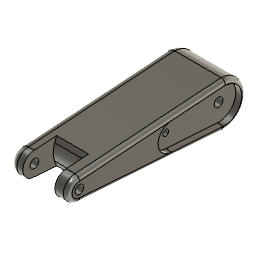
Assieme (Autodesk Fusion 360 archive; units mm, degrees)
design "Braccio cort"
Autodesk Fusion 360 part; units mm, degrees
sketch "Sketch1" plane through (0, 0, 0) normal (1, 0, 0) x (0, 1, 0)
  circle A0 centre (0, 0) radius 5.95
  line L0 (0, 0) -> (-18.2, 0)
  circle A1 centre (-18.2, 0) radius 4.7
  line L1 (-18.2, 4.7) -> (-0.412348, 5.935694)
  line L2 (-18.2, -4.7) -> (-0.412348, -5.935694)
  line L3 (0, 0) -> (-50, 0)
  circle A2 centre (-50, 0) radius 1.5
  circle A3 centre (0, 0) radius 7.5
  circle A4 centre (-50, 0) radius 4
  line L4 (-50.000001, 4) -> (0.297212, 7.494109)
  line L5 (-50.000001, -4) -> (-0.52648, -7.481498)
  circle A5 centre (0, 0) radius 1.5
  dimension "d1" = 11.9
  dimension "d2" = 18.2
  dimension "d3" = 9.4
  dimension "d4" = 50
  dimension "d5" = 3
  dimension "d6" = 15
  dimension "d7" = 8
  dimension "d12" = 3
  constraint coincident A0.centre L0.start
  constraint horizontal L0
  constraint coincident L0.end A1.centre
  constraint coincident A1 L1.start
  constraint tangent A0 L1
  constraint coincident A1 L2.start
  constraint tangent A0 L2
  constraint parallel L0 L3
  constraint coincident L3.end A2.centre
  constraint concentric A0 A3
  constraint concentric A2 A4
  constraint parallel L1 L4
  constraint tangent A3 L5
  constraint concentric A3 A5
  measures "d1" diameter of A0
  measures "d2" distance of A0.centre L0.end
  measures "d3" diameter of A1
  measures "d4" distance of A0.centre L3.end
  measures "d5" diameter of A2
  measures "d6" diameter of A3
  measures "d7" diameter of A4
  measures "d12" diameter of A5
extrude "Extrude1" add sketch "Sketch1" against normal blind 20 contours A0 | A0 L1 L2 A3 L4 | A0 L0 L1 L3 A3 | A0 L0 L2 L3 A3 | L0 A1 L1 L3 A3 | A1 L1 L3 A3 A4 L4 | A1 L2 L3 A3 A4 L5 | L0 A1 L2 L3 A3 | L0 A1 L3 | L0 A1 L3 | A4 | A2 | A5 picked at (0.057913, 4.454197) picked at (-0.481904, 6.936944) picked at (-4.913133, 4.943319) picked at (-4.913133, -4.943319) picked at (-9.491083, 0.574667) picked at (-23.269385, 5.029406) picked at (-23.455372, -5.333731) picked at (-9.491083, -0.574667) picked at (-17.97704, 3.117387) picked at (-21.317387, -0.22296) picked at (-50.236089, -3.150376) picked at (-49.655688, 0.192709) picked at (0.715636, -0.549431)
extrude "Extrude2" cut sketch "Sketch1" against normal blind 2.05 contours A0 | A0 L0 L1 L3 A3 | A0 L0 L2 L3 A3 | L0 A1 L1 L3 A3 | L0 A1 L2 L3 A3 | L0 A1 L3 | L0 A1 L3 | A5 picked at (0.057913, 4.454197) picked at (-4.913133, 4.943319) picked at (-4.913133, -4.943319) picked at (-9.491083, 0.574667) picked at (-9.491083, -0.574667) picked at (-17.97704, 3.117387) picked at (-21.317387, -0.22296) picked at (0.715636, -0.549431)
extrude "Extrude3" cut sketch "Sketch1" against normal through all contours A2 | A5 picked at (-49.655688, 0.192709) picked at (0.715636, -0.549431)
sketch "Sketch2" plane through (-20, 0, 0) normal (-1, 0, 0) x (0, -1, 0)
  arc A0 (50.000001, -4) -> (50.000001, 4) centre (50, 0) ccw
  line L0 (50.000001, 4) -> (-0.297212, 7.494109)
  arc A1 (-0.297212, 7.494109) -> (0.52648, -7.481498) centre (0, 0) ccw
  line L1 (0.52648, -7.481498) -> (50.000001, -4)
  circle A2 centre (0, 0) radius 3
  circle A3 centre (0, 0) radius 1.5
  circle A4 centre (50, 0) radius 1.5
  dimension "d15" = 6
  measures "d15" diameter of A2
extrude "Extrude4" cut sketch "Sketch2" against normal blind 10 contours A2 | A3 picked at (2.488831, -0.149042) picked at (0.56701, -0.538293)
sketch "Sketch3" plane through (0, 0, 0) normal (1, 0, 0) x (0, 1, 0)
  circle A0 centre (-50.000001, 0) radius 6
  line L0 (-44.000001, 7) -> (-56.000001, 7)
  line L1 (-56.000001, 7) -> (-56.000001, -7)
  line L2 (-56.000001, -7) -> (-44.000001, -7)
  line L3 (-44.000001, -7) -> (-44.000001, 7)
  line L4 (-44.000001, 7) -> (-56.000001, -7) construction
  line L5 (-56.000001, 7) -> (-44.000001, -7) construction
  line L6 (-44.000001, 0) -> (-40.579799, 9.396926)
  line L7 (-44.000001, 0) -> (-34.000001, 0) construction
  line L8 (-44.000001, 7) -> (-39.000001, 7)
  line L9 (-50.000001, 0) -> (-39.000001, 0)
  line L10 (-44.000001, -7) -> (-39.000001, -7)
  line L11 (-44.000001, 0) -> (-40.579799, -9.396926)
  point P0 (-50.000001, 0)
  dimension "d18" = 12
  dimension "d22" = 70
  dimension "d23" = 10
  constraint horizontal L0
  constraint perpendicular L0 L1
  constraint parallel L0 L2
  constraint parallel L1 L3
  constraint horizontal L7
  constraint perpendicular L3 L8
  measures "d18" diameter of A0
  measures "d22" angle of L6 L7
extrude "Extrude5" cut sketch "Sketch3" along normal mid plane 11 from surface at -10 contours A0 | A0 L1 L2 L3 | L3 L10 L11 | A0 L0 L1 L3 | L3 L6 L8 picked at (-50.136181, 1.817196) picked at (-50.149461, -6.661074) picked at (-43.150737, -4.666667) picked at (-50.149461, 6.661074) picked at (-43.150737, 4.666667)
sketch "Sketch4" plane through (-2.05, 0, 0) normal (1, 0, 0) x (0, 1, 0)
  circle A0 centre (0, 0) radius 1.5
  arc A1 (-18.2, 4.7) -> (-18.2, -4.7) centre (-18.2, 0) ccw
  line L0 (-18.2, -4.7) -> (-0.412348, -5.935694)
  arc A2 (-0.412348, -5.935694) -> (-0.412348, 5.935694) centre (0, 0) ccw
  line L1 (-0.412348, 5.935694) -> (-18.2, 4.7)
  circle A3 centre (-18.2, 0) radius 4.7
  circle A4 centre (-18.2, 0) radius 1
  dimension "d24" = 2
  constraint concentric A1 A3
  constraint concentric A3 A4
  measures "d24" diameter of A4
extrude "Extrude6" cut sketch "Sketch4" against normal blind 9 contours A4 picked at (-18.12804, 0.310291)
fillet "Fillet1" radius 8 1 edges at (-10, -44.000001, 0)
fillet "Fillet2" radius 2.5 4 edges at (-20, -24.851395, 5.747054) (-20, 7.488681, -0.411894) (-20, -25.26324, -5.740749) (-20, -54, 0)
fillet "Fillet2" radius 1.5 4 edges at (0, -24.851395, 5.747054) (0, -25.26324, -5.740749) (0, 7.488681, -0.411894) (0, -54, 0)

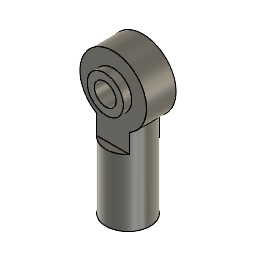
design "M3 angolare"
Autodesk Fusion 360 part; units mm, degrees
sketch "Sketch1" plane through (0, 0, 0) normal (0, 0, 1) x (1, 0, 0)
  circle A0 centre (0, 0) radius 3
  dimension "d6" = 6
  constraint coincident A0.centre origin
  measures "d6" diameter of A0
extrude "Extrude1" add sketch "Sketch1" along normal blind 15.5 makes body 1
sketch "Sketch3" plane through (0, 0, 0) normal (0, 1, 0) x (1, 0, 0)
  line L0 (0, 0) -> (0, -15.5)
  circle A0 centre (0, -15.5) radius 4.5
  circle A1 centre (0, -15.5) radius 2.5
  dimension "d5" = 9
  dimension "d9" = 5
  constraint coincident L0.start origin
  constraint vertical L0
  constraint coincident L0.end A0.centre
  constraint concentric A0 A1
  measures "d5" diameter of A0
  measures "d9" diameter of A1
extrude "Extrude2" add sketch "Sketch3" along normal mid plane 6 contours A0 | A1 bodies 1
extrude "Extrude3" cut sketch "Sketch3" along normal mid plane 6 contours A1 bodies 1
sketch "Sketch4" plane through (0, 0, 0) normal (1, 0, 0) x (0, 1, 0)
  line L0 (0, 20) -> (2, 20)
  line L1 (2, 20) -> (-2, 20)
  line L2 (-2, 20) -> (-2, 9)
  line L3 (-2, 9) -> (2, 9)
  line L4 (2, 9) -> (2, 20)
  line L5 (-3, 20) -> (3, 20)
  line L6 (3, 20) -> (3, 9)
  line L7 (3, 9) -> (-3, 9)
  line L8 (-3, 9) -> (-3, 20)
  dimension "d12" = 2
  dimension "d13" = 4
  dimension "d14" = 11
  constraint horizontal L0
  constraint horizontal L1
  constraint vertical L2
  constraint horizontal L3
  constraint vertical L4
  constraint horizontal L5
  constraint vertical L6
  constraint horizontal L7
  constraint vertical L8
  measures "d12" distance of L0.start L0.end
  measures "d13" distance of L0.end L1.end
  measures "d14" distance of L0.end L3.end
extrude "Extrude4" cut sketch "Sketch4" along normal mid plane 10 contours L4 L5 L6 L7 | L2 L5 L7 L8 bodies 1
sketch "Sketch5" plane through (0, 0, 0) normal (1, 0, 0) x (0, 1, 0)
  circle A0 centre (-10.5, -7) radius 2.5
  circle A1 centre (-10.5, -7) radius 1.5
  dimension "d19" = 5
  dimension "d20" = 3
  constraint concentric A0 A1
  measures "d19" diameter of A0
  measures "d20" diameter of A1
extrude "Extrude5" add sketch "Sketch5" along normal blind 6 separate body makes body 2
copy_body "Body->Comp1" bodies 1 removing the originals makes body 3 in component "Component"
copy_body "Body->Comp2" bodies 2 removing the originals makes body 4 in component "Component'"
component "Component" placed x (1, 0, 0) y (0, 1, 0) z (0, 0, 1) at (0, 0, 0)
component "Component'" placed x (0, -1, 0) y (1, 0, 0) z (0, 0, 1) at (10.5, 3, 22.5)
component "M3 angolare v1" placed x (1, 0, 0) y (0, 1, 0) z (0, 0, 1) at (0, 0, 0) in component "Component"
equation "d1 = 20 mm - 4.5 mm"

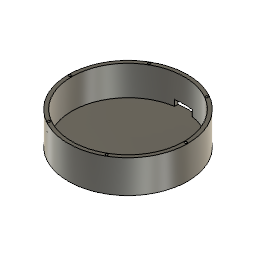
design "Base"
Autodesk Fusion 360 part; units mm, degrees
sketch "Sketch1" plane through (0, 0, 0) normal (0, 0, 1) x (1, 0, 0)
  circle A0 centre (0, 0) radius 100
  circle A1 centre (0, 0) radius 94
  dimension "d1" = 200
  dimension "d2" = -6
  constraint coincident A0.centre A1.centre
  measures "d1" diameter of A0
extrude "Extrude1" add sketch "Sketch1" along normal blind 50
sketch "Sketch2" plane through (0, 0, 50) normal (0, 0, 1) x (-1, 0, 0)
  circle A0 centre (0, 0) radius 94
  circle A1 centre (0, 0) radius 100
  circle A2 centre (0, 0) radius 94
  circle A3 centre (0, 0) radius 100
  circle A4 centre (0, 0) radius 97
  line L0 (0, 0) -> (115, 0)
  circle A5 centre (97, 0) radius 2
  dimension "d7" = 194
  dimension "d8" = 200
  dimension "d9" = 188
  dimension "d10" = 4
  constraint concentric A0 A2
  constraint coincident A0.centre A1.centre
  constraint horizontal L0
  constraint coincident A4 A5.centre
  constraint coincident L0 A5.centre
  measures "d7" diameter of A4
  measures "d8" diameter of A3
  measures "d9" diameter of A2
  measures "d10" diameter of A5
extrude "Extrude2" cut sketch "Sketch2" against normal blind 15 contours A4 L0 A5 | A4 L0 A5 | A4 L0 A5 | A4 L0 A5
pattern_circular "C-Pattern1" count 6 over 360 about axis through (0, 0, 1.75) along (0, 0, 1) of "Extrude2"
sketch "Sketch3" plane through (0, 0, 0) normal (0, 0, -1) x (1, 0, 0)
  circle A0 centre (0, 0) radius 94
  circle A1 centre (0, 0) radius 100
  circle A2 centre (0, 0) radius 100
  constraint concentric A0 A2
extrude "Extrude3" add sketch "Sketch3" along normal blind 5 contours A0 | A1 A2
sketch "Sketch4" plane through (0, 0, 0) normal (0, 1, 0) x (1, 0, 0)
  line L0 (0, 0) -> (15, 0)
  line L1 (15, 0) -> (15, -10)
  line L2 (15, -10) -> (0, -10)
  line L3 (0, -10) -> (0, 0)
  line L4 (0, 0) -> (-15, 0)
  line L5 (-15, 0) -> (-15, -10)
  line L6 (-15, -10) -> (0, -10)
  line L7 (0, -10) -> (0, 0)
  dimension "d17" = 15
  dimension "d18" = 10
  dimension "d19" = 10
  constraint horizontal L0
  constraint vertical L1
  constraint horizontal L2
  constraint vertical L3
  constraint coincident L0.start L3.end
  constraint horizontal L4
  constraint vertical L5
  constraint horizontal L6
  constraint vertical L7
  measures "d17" distance of L0.start L0.end
  measures "d18" distance of L0.start L2.end
  measures "d19" distance of L0.start L2.end
extrude "Extrude4" cut sketch "Sketch4" along normal blind 100
equation "d7 = d9 + ( ( d8 - d9 ) * 0.5 )"

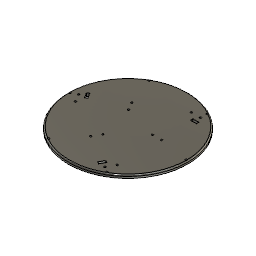
design "Senza titolo"
Autodesk Fusion 360 part; units mm, degrees
sketch "Schizzo1" plane through (0, 0, 0) normal (0, 0, 1) x (1, 0, 0)
  line L0 (0, 0) -> (0, 50)
  line L1 (0, 50) -> (0, 60.7)
  line L2 (0, 60.7) -> (37, 60.7)
  line L3 (37, 60.7) -> (37, 20.7)
  line L4 (37, 20.7) -> (0, 20.7)
  line L5 (0, 20.7) -> (0, 60.7)
  line L6 (-52.5677, -30.35) -> (-71.0677, 1.6929)
  line L7 (0, 0) -> (-43.3013, -25)
  line L8 (-36.4267, 21.6929) -> (-17.9267, -10.35)
  line L9 (-71.0677, 1.6929) -> (-36.4267, 21.6929)
  line L10 (-43.3013, -25) -> (-52.5677, -30.35)
  line L11 (-17.9267, -10.35) -> (-52.5677, -30.35)
  line L12 (52.5677, -30.35) -> (34.0677, -62.3929)
  line L13 (0, 0) -> (43.3013, -25)
  line L14 (-0.5733, -42.3929) -> (17.9267, -10.35)
  line L15 (34.0677, -62.3929) -> (-0.5733, -42.3929)
  line L16 (43.3013, -25) -> (52.5677, -30.35)
  line L17 (17.9267, -10.35) -> (52.5677, -30.35)
  circle A0 centre (0, 0) radius 100
  dimension "d1" = 50
  dimension "d2" = 10.7
  dimension "d3" = 37
  dimension "d4" = 40
  dimension "d6" = 360
  dimension "d7" = 200
  constraint coincident L0.start L7.start
  constraint vertical L0
  constraint parallel L0 L1
  constraint horizontal L2
  constraint vertical L3
  constraint horizontal L4
  constraint vertical L5
  measures "d1" distance of L0.start L0.end
  measures "d2" distance of L0.end L1.end
  measures "d3" distance of L1.end L2.end
  measures "d4" distance of L1.end L4.end
  measures "d7" diameter of A0
extrude "Estrusione1" add sketch "Schizzo1" along normal blind 10 contours L0 L1 L2 L3 L4 L5 | L6 L7 L8 L9 L10 L11 | L12 L13 L14 L15 L16 L17 | A0
sketch "Schizzo2" plane through (0, 0, 10) normal (0, 0, 1) x (-1, 0, 0)
  circle A0 centre (0, 0) radius 100
  line L0 (0, 0) -> (0, -50)
  line L1 (0, -50) -> (-32.95, -50)
  line L2 (-32.95, -50) -> (-32.95, -73.2)
  line L3 (-32.95, -73.2) -> (-47.95, -73.2)
  line L4 (-47.95, -73.2) -> (-47.95, -8.2)
  line L5 (-47.95, -8.2) -> (-32.95, -8.2)
  line L6 (-32.95, -8.2) -> (-32.95, -73.2)
  circle A1 centre (-32.95, -73.2) radius 1.5
  circle A2 centre (-32.95, -8.2) radius 1.5
  circle A3 centre (-47.95, -73.2) radius 1.5
  circle A4 centre (-47.95, -8.2) radius 1.5
  dimension "d33" = 50
  dimension "d34" = 32.95
  dimension "d35" = 23.2
  dimension "d36" = 15
  dimension "d37" = 65
  dimension "d38" = 3
  dimension "d39" = 3
  dimension "d40" = 3
  dimension "d41" = 3
  constraint coincident A0.centre L0.start
  constraint vertical L0
  constraint perpendicular L0 L1
  constraint perpendicular L1 L2
  constraint horizontal L3
  constraint vertical L4
  constraint horizontal L5
  constraint vertical L6
  constraint coincident L2.end L3.start
  constraint coincident L5.end L6.start
  constraint coincident L3.end L4.start
  constraint coincident L4.end L5.start
  measures "d33" distance of A0.centre L0.end
  measures "d34" distance of L0.end L1.end
  measures "d35" distance of L1.end L2.end
  measures "d36" distance of L2.end L3.end
  measures "d37" distance of L2.end L5.end
  measures "d38" diameter of A1
  measures "d39" diameter of A2
  measures "d40" diameter of A3
  measures "d41" diameter of A4
extrude "Extrude4" cut sketch "Schizzo2" against normal blind 60 contours L2 L3 L6 A1 | L2 L3 L6 A1 | L5 L6 A2 | L5 L6 A2 | L3 L4 A3 | L3 L4 A3 | L4 L5 A4 | L4 L5 A4
pattern_circular "C-Pattern2" count 3 over 360 about axis through (0, 0, 1.75) along (0, 0, 1) of "Extrude4"
sketch "Sketch4" plane through (0, 0, 10) normal (0, 0, 1) x (-1, 0, 0)
  circle A0 centre (0, 0) radius 100
  circle A1 centre (-32.95, -8.2) radius 1.5
  circle A2 centre (-32.95, -73.2) radius 1.5
  circle A3 centre (-47.95, -8.2) radius 1.5
  circle A4 centre (-47.95, -73.2) radius 1.5
  circle A5 centre (31.0764, -37.4259) radius 1.5
  circle A6 centre (79.8681, 8.0645) radius 1.5
  circle A7 centre (87.3681, -4.9259) radius 1.5
  circle A8 centre (23.5764, -24.4355) radius 1.5
  circle A9 centre (16.8736, 45.6259) radius 1.5
  circle A10 centre (-46.9181, 65.1355) radius 1.5
  circle A11 centre (-39.4181, 78.1259) radius 1.5
  circle A12 centre (9.3736, 32.6355) radius 1.5
  line L0 (-38.5766, 79.3677) -> (-31.6381, 75.3854)
  line L1 (-31.6381, 75.3854) -> (-34.6248, 70.1816)
  line L2 (-34.6248, 70.1816) -> (-31.1556, 68.1905)
  line L3 (-31.6381, 75.3854) -> (-28.1689, 73.3943)
  line L4 (-28.1689, 73.3943) -> (-31.1556, 68.1905)
  line L5 (-28.1689, 73.3943) -> (-26.1778, 76.8635)
  line L6 (-31.6381, 75.3854) -> (-29.647, 78.8547)
  line L7 (-29.647, 78.8547) -> (-26.1778, 76.8635)
  dimension "d46" = 8
  dimension "d47" = 6
  dimension "d48" = 4
  dimension "d49" = 4
  dimension "d54" = 4
  dimension "d55" = 4
  constraint coincident A11 L0.start
  constraint perpendicular L0 L1
  constraint perpendicular L1 L2
  constraint perpendicular L1 L3
  constraint perpendicular L3 L5
  constraint perpendicular L3 L6
  measures "d46" distance of L0.start L0.end
  measures "d47" distance of L0.end L1.end
  measures "d48" distance of L1.end L2.end
  measures "d49" distance of L0.end L3.end
  measures "d54" distance of L3.end L5.end
  measures "d55" distance of L0.end L6.end
extrude "Extrude5" cut sketch "Sketch4" against normal blind 40 contours L1 L2 L3 L4 | L3 L5 L6 L7
pattern_circular "C-Pattern3" count 3 over 360 about axis through (0, 0, -200) along (0, 0, 1) of "Extrude5"
extrude "Extrude6" cut 1 faces at (23.6749, -29.9689, 0) along direction (0, 0, 1) blind 5
sketch "Sketch5" plane through (0, 0, 10) normal (0, 0, 1) x (-1, 0, 0)
  line L0 (-31.1556, 68.1905) -> (-34.6248, 70.1816)
  line L1 (-34.6248, 70.1816) -> (-29.647, 78.8547)
  line L2 (-29.647, 78.8547) -> (-26.1778, 76.8635)
  line L3 (-26.1778, 76.8635) -> (-31.1556, 68.1905)
  circle A0 centre (0, 0) radius 100
  circle A1 centre (-32.95, -8.2) radius 1.5
  circle A2 centre (-32.95, -73.2) radius 1.5
  circle A3 centre (-47.95, -8.2) radius 1.5
  circle A4 centre (-47.95, -73.2) radius 1.5
  circle A5 centre (31.0764, -37.4259) radius 1.5
  circle A6 centre (79.8681, 8.0645) radius 1.5
  circle A7 centre (87.3681, -4.9259) radius 1.5
  circle A8 centre (23.5764, -24.4355) radius 1.5
  circle A9 centre (16.8736, 45.6259) radius 1.5
  circle A10 centre (-46.9181, 65.1355) radius 1.5
  circle A11 centre (-39.4181, 78.1259) radius 1.5
  circle A12 centre (9.3736, 32.6355) radius 1.5
  line L4 (-43.4769, -61.0768) -> (-43.4667, -65.0768)
  line L5 (-43.4667, -65.0768) -> (-53.4666, -65.1024)
  line L6 (-53.4666, -65.1024) -> (-53.4769, -61.1024)
  line L7 (-53.4769, -61.1024) -> (-43.4769, -61.0768)
  line L8 (74.6325, -7.1137) -> (78.0914, -5.1049)
  line L9 (78.0914, -5.1049) -> (83.1136, -13.7523)
  line L10 (83.1136, -13.7523) -> (79.6547, -15.7611)
  line L11 (79.6547, -15.7611) -> (74.6325, -7.1137)
  circle A13 centre (0, 0) radius 97
  line L12 (0, 0) -> (97, 0)
  circle A14 centre (97, 0) radius 1.5
  dimension "d60" = 194
  dimension "d61" = 3
  constraint coincident A0.centre A13.centre
  constraint coincident A13 L12.end
  constraint horizontal L12
  constraint coincident L12.end A14.centre
  measures "d60" diameter of A13
  measures "d61" diameter of A14
extrude "Extrude7" cut sketch "Sketch5" against normal blind 9.5 contours A13 L12 A14 | A13 A14 | A13 L12 A14 picked at (97.4791, 0.3082)
pattern_circular "C-Pattern4" count 6 over 360 about axis through (0, 0, 1.75) along (0, 0, 1) of "Extrude7"
fillet "Fillet2" radius 2 1 edges at (-93.2327, -36.1615, 10)
equation "d34 = 25 mm + 2.95 mm + 5 mm"
equation "d48 = d49"

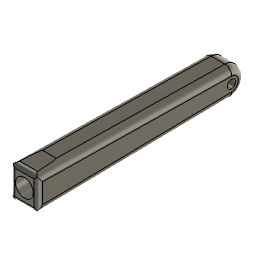
design "Braccio lungo"
Autodesk Fusion 360 part; units mm, degrees
sketch "Sketch1" plane through (0, 0, 0) normal (1, 0, 0) x (0, 1, 0)
  circle A0 centre (0, 0) radius 5
  circle A1 centre (0, 0) radius 1.5
  line L0 (0, 0) -> (-61, 0)
  line L1 (-61, -3.25) -> (-61, 3.25)
  line L2 (-61, -6) -> (-61, 6)
  line L3 (-61, 6) -> (0.081901, 4.999329)
  line L4 (-61, -6) -> (0.081901, -4.999329)
  dimension "d1" = 10
  dimension "d2" = 3
  dimension "d3" = 61
  dimension "d4" = 6.5
  dimension "d5" = 12
  constraint coincident A0.centre A1.centre
  constraint horizontal L0
  constraint midpoint L0.end L1
  constraint perpendicular L0 L1
  constraint midpoint L0.end L2
  constraint perpendicular L0 L2
  constraint tangent A0 L3
  constraint tangent A0 L4
  measures "d1" diameter of A0
  measures "d2" diameter of A1
  measures "d3" distance of A0.centre L0.end
  measures "d4" distance of L1.start L1.end
  measures "d5" distance of L2.start L2.end
extrude "Extrude1" add sketch "Sketch1" along normal mid plane 10 contours A0 | A0 L0 L1 L2 L3 | A0 L0 L1 L2 L4 picked at (-0.222664, -3.818097) picked at (-42.333333, 1.083333) picked at (-42.333333, -1.083333)
ref_plane "WorkPlane1" through (0, -61, 0) normal (0, 1, 0) x (0, 0, 1)
sketch "Sketch2" plane through (0, -61, 0) normal (0, 1, 0) x (1, 0, 0)
  circle A0 centre (0, 0) radius 3.25
  circle A1 centre (0, 0) radius 6
  line L0 (-5, -6) -> (5, -6)
  line L1 (5, -6) -> (5, 6)
  line L2 (5, 6) -> (-5, 6)
  line L3 (-5, 6) -> (-5, -6)
  line L4 (-5, -6) -> (5, 6) construction
  line L5 (5, -6) -> (-5, 6) construction
  dimension "d9" = 6.5
  dimension "d10" = 12
  constraint coincident A0.centre A1.centre
  constraint concentric A0 A1
  constraint horizontal L0
  constraint perpendicular L0 L1
  constraint parallel L0 L2
  constraint parallel L1 L3
  constraint coincident L4 A0.centre
  constraint coincident L5 A0.centre
  measures "d9" diameter of A0
  measures "d10" diameter of A1
extrude "Extrude2" add sketch "Sketch2" against normal blind 9 contours A1 L1 L3 | A1 L1 L2 | A1 L0 L1 | A1 L2 L3 | A1 L0 L3 picked at (4.416667, 0) picked at (4.027994, 5.216371) picked at (4.027994, -5.216371) picked at (-4.027994, 5.216371) picked at (-4.027994, -5.216371)
sketch "Sketch3" plane through (0, -61, 0) normal (0, -1, 0) x (1, 0, 0)
  circle A0 centre (0, 0) radius 3.25
  circle A1 centre (0, 0) radius 1.5
  dimension "d13" = 3
  constraint coincident A0.centre A1.centre
  measures "d13" diameter of A1
extrude "Extrude3" cut sketch "Sketch3" against normal blind 6 contours A1 picked at (0.56701, -0.538293)
sketch "Sketch4" plane through (-5, 0, 0) normal (-1, 0, 0) x (0, -1, 0)
  circle A0 centre (0, 0) radius 1.5
  line L0 (61, 6) -> (-0.081901, 4.999329)
  arc A1 (-0.081901, 4.999329) -> (-0.081901, -4.999329) centre (0, 0) ccw
  line L1 (-0.081901, -4.999329) -> (61, -6)
  line L2 (61, -6) -> (70, -6)
  line L3 (70, -6) -> (70, 6)
  line L4 (70, 6) -> (61, 6)
  line L5 (70, 0) -> (57, 0)
  line L6 (57, 0) -> (57, 3)
  line L7 (57, 3) -> (32, 3)
  line L8 (32, 3) -> (32, -3)
  line L9 (32, -3) -> (57, -3)
  line L10 (57, -3) -> (57, 3)
  dimension "d16" = 13
  dimension "d17" = 3
  dimension "d18" = 25
  dimension "d19" = 6
  constraint midpoint L3 L5.start
  constraint perpendicular L3 L5
  constraint perpendicular L5 L6
  constraint horizontal L7
  constraint vertical L8
  constraint horizontal L9
  constraint vertical L10
  measures "d16" distance of L5.start L5.end
  measures "d17" distance of L5.end L6.end
  measures "d18" distance of L6.end L7.end
  measures "d19" distance of L6.end L9.end
extrude "Extrude4" cut sketch "Sketch4" against normal blind 7 contours L6 L7 L8 L9 L10 picked at (40.333333, 0)
fillet "Fillet1" radius 1.5 4 edges at (-5, -70, 0) (0, -70, 6) (5, -70, 0) (0, -70, -6)
fillet "Fillet2" radius 2.5 6 edges at (-5, -30.459049, 5.499665) (-5, 5, 0) (-5, -30.459049, -5.499665) (5, -30.459049, -5.499665) (5, 5, 0) (5, -30.459049, 5.499665)
chamfer "Chamfer1" distance 14 distance2 5 1 edges at (-5, -32, 0) measured on face at (-5, -21.833333, 0)
sketch "Sketch5" plane through (2, 0, 0) normal (-1, 0, 0) x (0, -1, 0)
  line L0 (57, -3) -> (57, 3)
  line L1 (57, 3) -> (32, 3)
  line L2 (32, 3) -> (32, -3)
  line L3 (32, -3) -> (57, -3)
  line L4 (57, -3) -> (54, -3)
  line L5 (54, -3) -> (54, 3)
  line L6 (54, 3) -> (57, 3)
  line L7 (57, 3) -> (57, -3)
  dimension "d28" = 3
  dimension "d29" = 6
  constraint horizontal L4
  constraint vertical L5
  constraint horizontal L6
  constraint vertical L7
  constraint coincident L0.start L3.end
  measures "d28" distance of L0.start L4.end
  measures "d29" distance of L0.start L0.end
extrude "Extrude5" cut sketch "Sketch5" against normal blind 1 contours L0 L1 L3 L4 L5 L6 L7 picked at (55, 1)

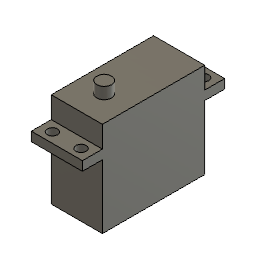
design "Motore"
Autodesk Fusion 360 part; units mm, degrees
sketch "Schizzo1" plane through (0, 0, 0) normal (0, 1, 0) x (1, 0, 0)
  line L0 (0, 0) -> (20, 0)
  line L1 (20, 0) -> (20, 40)
  line L2 (20, 40) -> (0, 40)
  line L3 (0, 40) -> (0, 0)
  dimension "d1" = 20
  dimension "d2" = 40
  constraint horizontal L0
  constraint vertical L1
  constraint horizontal L2
  constraint vertical L3
  constraint coincident L0.start L3.end
  measures "d1" distance of L0.start L0.end
  measures "d2" distance of L0.start L2.end
extrude "Estrusione1" add sketch "Schizzo1" along normal blind 25
sketch "Schizzo2" plane through (0, 25, 0) normal (0, 1, 0) x (-1, 0, 0)
  line L0 (0, -40) -> (0, 0)
  line L1 (0, 0) -> (-20, 0)
  line L2 (-20, 0) -> (-20, -40)
  line L3 (-20, -40) -> (0, -40)
  line L4 (0, -40) -> (0, -47.8)
  line L5 (0, -47.8) -> (-20, -47.8)
  line L6 (-20, -47.8) -> (-20, 7.8)
  line L7 (-20, 7.8) -> (0, 7.8)
  line L8 (0, 7.8) -> (0, -47.8)
  dimension "d5" = 7.8
  dimension "d6" = 55.6
  constraint coincident L0.start L3.end
  constraint perpendicular L3 L4
  constraint horizontal L5
  constraint vertical L6
  constraint horizontal L7
  constraint vertical L8
  measures "d5" distance of L0.start L4.end
  measures "d6" distance of L4.end L7.end
extrude "Estrusione2" add sketch "Schizzo2" along normal blind 3.6
sketch "Schizzo3" plane through (0, 28.6, 0) normal (0, 1, 0) x (-1, 0, 0)
  line L0 (0, 7.8) -> (-20, 7.8)
  line L1 (-20, 7.8) -> (-20, -47.8)
  line L2 (-20, -47.8) -> (0, -47.8)
  line L3 (0, -47.8) -> (0, 7.8)
  line L4 (0, -47.8) -> (-20, -47.8)
  line L5 (-20, -47.8) -> (-20, -40)
  line L6 (-20, -40) -> (0, -40)
  line L7 (0, -40) -> (0, -47.8)
  line L8 (0, 7.8) -> (-20, 7.8)
  line L9 (-20, 7.8) -> (-20, 0)
  line L10 (-20, 0) -> (0, 0)
  line L11 (0, 0) -> (0, 7.8)
  dimension "d9" = 20
  dimension "d10" = 7.8
  dimension "d11" = 7.8
  constraint horizontal L4
  constraint vertical L5
  constraint horizontal L6
  constraint vertical L7
  constraint coincident L2.end L3.start
  constraint horizontal L8
  constraint vertical L9
  constraint horizontal L10
  constraint vertical L11
  constraint coincident L0.start L3.end
  measures "d9" distance of L2.end L1.end
  measures "d10" distance of L2.end L6.end
  measures "d11" distance of L0.start L10.end
extrude "Estrusione3" add sketch "Schizzo3" along normal blind 8.4 contours L1 L3 L6 L10
sketch "Schizzo4" plane through (0, 37, 0) normal (0, 1, 0) x (-1, 0, 0)
  line L0 (-20, -40) -> (0, -40)
  line L1 (0, -40) -> (0, 0)
  line L2 (0, 0) -> (-20, 0)
  line L3 (-20, 0) -> (-20, -40)
  line L4 (-10, 0) -> (-10, -13.6)
  circle A0 centre (-10, -10.7) radius 2.9
  dimension "d14" = 13.6
  dimension "d17" = 5.8
  dimension "d18" = 2.9
  constraint midpoint L2 L4.start
  constraint perpendicular L2 L4
  constraint coincident L4 A0.centre
  measures "d14" distance of L4.start L4.end
  measures "d17" diameter of A0
  measures "d18" distance of L4.end A0.centre
extrude "Estrusione4" add sketch "Schizzo4" along normal blind 4.5 contours L4 A0 | L4 A0
ref_plane "WorkPlane1" through (10, 0, 0) normal (1, 0, 0) x (0, 1, 0)
sketch "Sketch5" plane through (10, 0, 0) normal (1, 0, 0) x (0, 1, 0)
  line L0 (0, 0) -> (0, -10.7)
  line L1 (0, -10.7) -> (1, -10.7)
  line L2 (1, -10.7) -> (37, -10.7)
  line L3 (37, -10.7) -> (41.5, -10.7)
  dimension "d22" = 10.7
  dimension "d23" = 4.5
  constraint coincident L0.start origin
  constraint vertical L0
  constraint perpendicular L0 L1
  constraint perpendicular L0 L2
  constraint perpendicular L0 L3
  measures "d22" distance of L0.start L0.end
  measures "d23" distance of L2.end L3.end
sketch "Schizzo6" plane through (0, 28.6, 0) normal (0, 1, 0) x (-1, 0, 0)
  line L0 (-20, 0) -> (0, 0)
  line L1 (0, 0) -> (0, 7.8)
  line L2 (0, 7.8) -> (-20, 7.8)
  line L3 (-20, 7.8) -> (-20, 0)
  circle A0 centre (-4.4, 3.9) radius 2
  circle A1 centre (-15.6, 3.9) radius 2
  dimension "d24" = 4
  dimension "d26" = 4.4
  dimension "d27" = 3.9
  dimension "d28" = 4
  dimension "d29" = 4.4
  dimension "d30" = 3.9
  measures "d24" diameter of A0
  measures "d26" distance of L1 A0.centre
  measures "d27" distance of L2 A0.centre
  measures "d28" diameter of A1
  measures "d29" distance of L3 A1.centre
  measures "d30" distance of L2 A1.centre
extrude "Estrusione5" cut sketch "Schizzo6" against normal blind 20 contours A0 | A1
sketch "Schizzo7" plane through (0, 28.6, 0) normal (0, 1, 0) x (-1, 0, 0)
  line L0 (0, -40) -> (-20, -40)
  line L1 (-20, -40) -> (-20, -47.8)
  line L2 (-20, -47.8) -> (0, -47.8)
  line L3 (0, -47.8) -> (0, -40)
  circle A0 centre (-4.4, -43.9) radius 2
  circle A1 centre (-15.6, -43.9) radius 2
  dimension "d34" = 4
  dimension "d35" = 4
  dimension "d36" = 4.4
  dimension "d37" = 4.4
  dimension "d38" = 3.9
  dimension "d39" = 3.9
  measures "d34" diameter of A0
  measures "d35" diameter of A1
  measures "d36" distance of L3 A0.centre
  measures "d37" distance of L1 A1.centre
  measures "d38" distance of L2 A1.centre
  measures "d39" distance of L2 A0.centre
extrude "Estrusione6" cut sketch "Schizzo7" against normal blind 10 contours A0 | A1
sketch "Sketch9" plane through (0, 28.6, 0) normal (0, 1, 0) x (-1, 0, 0)
  circle A0 centre (-4.4, 3.9) radius 2
  circle A1 centre (-15.6, 3.9) radius 2
  line L0 (-20, 0) -> (0, 0)
  line L1 (0, 0) -> (0, 7.8)
  line L2 (0, 7.8) -> (-20, 7.8)
  line L3 (-20, 7.8) -> (-20, 0)
  line L4 (0, 7.8) -> (-20, 7.8)
  line L5 (-20, 7.8) -> (-20, -47.8)
  line L6 (-20, -47.8) -> (0, -47.8)
  line L7 (0, -47.8) -> (0, 7.8)
  line L8 (-10, -47.8) -> (-10, 7.8)
  line L9 (-20, -20) -> (0, -20)
  line L10 (-15.6, 3.9) -> (-4.4, 3.9)
  circle A2 centre (-15.6, 3.9) radius 2
  dimension "d42" = 23.9
  dimension "d43" = 11.2
  dimension "d44" = 27.8
  dimension "d45" = 20
  constraint horizontal L4
  constraint vertical L5
  constraint horizontal L6
  constraint vertical L7
  constraint coincident L1.end L2.start
  constraint midpoint L6 L8.start
  constraint midpoint L2 L8.end
  constraint midpoint L5 L9.start
  constraint midpoint L7 L9.end
  constraint coincident A1.centre L10.start
  constraint coincident A0.centre L10.end
  measures "d42" distance of L9 L10
  measures "d43" distance of A1.centre A0.centre
  measures "d44" distance of L4 L9
  measures "d45" distance of L5 L7
equation "d26 = 2.40 mm + 2 mm"
equation "d27 = 5.9 mm - 2 mm"

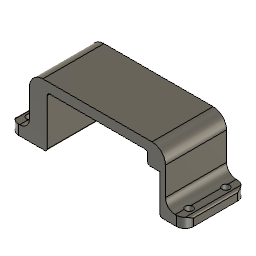
design "v2"
Autodesk Fusion 360 part; units mm, degrees
sketch "Sketch1" plane through (0, 0, 0) normal (0, 1, 0) x (1, 0, 0)
  line L0 (20.5, -10.5) -> (-20.5, -10.5)
  line L1 (-20.5, -10.5) -> (-20.5, 10.5)
  line L2 (-20.5, 10.5) -> (20.5, 10.5)
  line L3 (20.5, 10.5) -> (20.5, -10.5)
  line L4 (20.5, -10.5) -> (-20.5, 10.5) construction
  line L5 (-20.5, -10.5) -> (20.5, 10.5) construction
  line L6 (-23.9, -5.6) -> (23.9, -5.6)
  line L7 (23.9, -5.6) -> (23.9, 5.6)
  line L8 (23.9, 5.6) -> (-23.9, 5.6)
  line L9 (-23.9, 5.6) -> (-23.9, -5.6)
  line L10 (-23.9, -5.6) -> (23.9, 5.6) construction
  line L11 (23.9, -5.6) -> (-23.9, 5.6) construction
  circle A0 centre (-23.9, -5.6) radius 2
  circle A1 centre (-23.9, 5.6) radius 2
  circle A2 centre (23.9, -5.6) radius 2
  circle A3 centre (23.9, 5.6) radius 2
  line L12 (-27.8, 10.5) -> (27.8, 10.5)
  line L13 (27.8, 10.5) -> (27.8, -10.5)
  line L14 (27.8, -10.5) -> (-27.8, -10.5)
  line L15 (-27.8, -10.5) -> (-27.8, 10.5)
  line L16 (-27.8, 10.5) -> (27.8, -10.5) construction
  line L17 (27.8, 10.5) -> (-27.8, -10.5) construction
  line L18 (-27.8, -10.5) -> (27.8, -10.5)
  line L19 (27.8, -10.5) -> (27.8, -14.5)
  line L20 (27.8, -14.5) -> (-27.8, -14.5)
  line L21 (-27.8, -14.5) -> (-27.8, -10.5)
  line L22 (-27.8, 10.5) -> (-35.8, 10.5)
  line L23 (-35.8, 10.5) -> (-35.8, 6.5)
  line L24 (-35.8, 6.5) -> (-27.8, 6.5)
  line L25 (-27.8, 6.5) -> (-27.8, 10.5)
  line L26 (27.8, 10.5) -> (35.8, 10.5)
  line L27 (35.8, 10.5) -> (35.8, 6.5)
  line L28 (35.8, 6.5) -> (27.8, 6.5)
  line L29 (27.8, 6.5) -> (27.8, 10.5)
  dimension "d17" = 41
  dimension "d18" = 21
  dimension "d19" = 47.8
  dimension "d20" = 11.2
  dimension "d21" = 4
  dimension "d22" = 4
  dimension "d23" = 4
  dimension "d24" = 4
  dimension "d25" = 55.6
  dimension "d26" = 21
  dimension "d27" = 55.6
  dimension "d28" = 4
  dimension "d29" = 8
  dimension "d30" = 4
  dimension "d31" = 8
  dimension "d32" = 4
  constraint horizontal L0
  constraint perpendicular L0 L1
  constraint parallel L0 L2
  constraint parallel L1 L3
  constraint coincident L4 origin
  constraint coincident L5 origin
  constraint horizontal L6
  constraint perpendicular L6 L7
  constraint parallel L6 L8
  constraint parallel L7 L9
  constraint coincident L10 origin
  constraint coincident L11 origin
  constraint coincident L6.start L9.end
  constraint coincident L8.end L9.start
  constraint coincident L6.end L7.start
  constraint coincident L7.end L8.start
  constraint horizontal L12
  constraint perpendicular L12 L13
  constraint parallel L12 L14
  constraint parallel L13 L15
  constraint coincident L16 origin
  constraint coincident L17 origin
  constraint horizontal L18
  constraint vertical L19
  constraint horizontal L20
  constraint vertical L21
  constraint horizontal L22
  constraint vertical L23
  constraint horizontal L24
  constraint vertical L25
  constraint horizontal L26
  constraint vertical L27
  constraint horizontal L28
  constraint vertical L29
  measures "d17" distance of L1.end L2.end
  measures "d18" distance of L0.end L1.end
  measures "d19" distance of L7.end L8.end
  measures "d20" distance of L6.end L7.end
  measures "d21" diameter of A0
  measures "d22" diameter of A1
  measures "d23" diameter of A2
  measures "d24" diameter of A3
  measures "d25" distance of L13.end L14.end
  measures "d26" distance of L12.end L13.end
  measures "d27" distance of L14.end L13.end
  measures "d28" distance of L14.end L20.end
  measures "d29" distance of L12.start L22.end
  measures "d30" distance of L12.start L24.end
  measures "d31" distance of L12.end L26.end
  measures "d32" distance of L12.end L28.end
extrude "Extrude1" add sketch "Sketch1" along normal blind 25 contours L0 L14 L18 L19 L20 L21 | L3 L6 L7 L8 A2 A3 L12 L13 L14 L18 L29 | L1 L6 L8 L9 A0 A1 L12 L14 L15 L18 L25 | L3 L6 L7 L8 A2 A3 | L1 L6 L8 L9 A0 A1 | L13 L26 L27 L28 L29 | L15 L22 L23 L24 L25
sketch "Sketch2" plane through (0, 0, -6.5) normal (0, 0, 1) x (-1, 0, 0)
  line L0 (-27.8, 0) -> (-35.8, 0)
  line L1 (-35.8, 0) -> (-35.8, -25)
  line L2 (-35.8, -25) -> (-27.8, -25)
  line L3 (-27.8, -25) -> (-27.8, 0)
  line L4 (0, 0) -> (0, -25)
  line L5 (32.5, -5) -> (-32.5, -5)
  line L6 (-32.5, -5) -> (-32.5, -20)
  line L7 (-32.5, -20) -> (32.5, -20)
  line L8 (32.5, -20) -> (32.5, -5)
  line L9 (32.5, -5) -> (-32.5, -20) construction
  line L10 (-32.5, -5) -> (32.5, -20) construction
  circle A0 centre (32.5, -20) radius 1.5
  circle A1 centre (32.5, -5) radius 1.5
  circle A2 centre (-32.5, -20) radius 1.5
  circle A3 centre (-32.5, -5) radius 1.5
  point P0 (0, -12.5)
  dimension "d35" = 65
  dimension "d36" = 15
  dimension "d37" = 3
  dimension "d38" = 3
  dimension "d39" = 3
  dimension "d40" = 3
  constraint coincident L4.start origin
  constraint vertical L4
  constraint horizontal L5
  constraint perpendicular L5 L6
  constraint parallel L5 L7
  constraint parallel L6 L8
  constraint coincident L9 P0
  constraint coincident L10 P0
  constraint midpoint L4 P0
  constraint coincident L7.end L8.start
  constraint coincident L5.start L8.end
  constraint coincident L6.end L7.start
  constraint coincident L5.end L6.start
  measures "d35" distance of L6.end L7.end
  measures "d36" distance of L5.end L6.end
  measures "d37" diameter of A0
  measures "d38" diameter of A1
  measures "d39" diameter of A2
  measures "d40" diameter of A3
extrude "Extrude2" cut sketch "Sketch2" against normal blind 12 contours L5 L6 A3 | L5 L6 A3 | L6 L7 A2 | L6 L7 A2 | L5 L8 A1 | L5 L8 A1 | L7 L8 A0 | L7 L8 A0
fillet "Fillet1" radius 4 2 edges at (27.8, 12.5, -6.5) (-27.8, 12.5, -6.5)
fillet "Fillet2" radius 5.5 2 edges at (-27.8, 12.5, 14.5) (27.8, 12.5, 14.5)
extrude "Extrude3" add sketch "Sketch1" along normal blind 15 contours L6 L7 A2 | L6 L7 A2 | L6 L9 A0 | L6 L9 A0 | L7 L8 A3 | L7 L8 A3 | L8 L9 A1 | L8 L9 A1
sketch "Sketch3" plane through (0, 0, 0) normal (0, -1, 0) x (1, 0, 0)
  arc A0 (27.8, 9) -> (22.3, 14.5) centre (22.3, 9) ccw
  line L0 (22.3, 14.5) -> (-22.3, 14.5)
  arc A1 (-22.3, 14.5) -> (-27.8, 9) centre (-22.3, 9) ccw
  line L1 (-27.8, 9) -> (-27.8, -2.5)
  arc A2 (-31.8, -6.5) -> (-27.8, -2.5) centre (-31.8, -2.5) ccw
  line L2 (-31.8, -6.5) -> (-35.8, -6.5)
  line L3 (-35.8, -6.5) -> (-35.8, -10.5)
  line L4 (-35.8, -10.5) -> (-20.5, -10.5)
  line L5 (-20.5, -10.5) -> (-20.5, 10.5)
  line L6 (-20.5, 10.5) -> (20.5, 10.5)
  line L7 (20.5, 10.5) -> (20.5, -10.5)
  line L8 (20.5, -10.5) -> (35.8, -10.5)
  line L9 (35.8, -10.5) -> (35.8, -6.5)
  line L10 (35.8, -6.5) -> (31.8, -6.5)
  arc A3 (27.8, -2.5) -> (31.8, -6.5) centre (31.8, -2.5) ccw
  line L11 (27.8, -2.5) -> (27.8, 9)
  line L12 (-20.5, -10.5) -> (-25.5, -10.5)
  line L13 (-25.5, -10.5) -> (-25.5, 5.5)
  line L14 (-25.5, 5.5) -> (-20.5, 5.5)
  line L15 (-20.5, 5.5) -> (-20.5, -10.5)
  line L16 (0, 0) -> (0, -3)
  line L17 (20.5, -10.5) -> (25.5, -10.5)
  line L18 (25.5, -10.5) -> (25.5, 5.5)
  line L19 (25.5, 5.5) -> (20.5, 5.5)
  line L20 (20.5, 5.5) -> (20.5, -10.5)
  dimension "d45" = 5
  dimension "d46" = 16
  dimension "d47" = 5
  dimension "d48" = 16
  constraint horizontal L12
  constraint vertical L13
  constraint horizontal L14
  constraint vertical L15
  constraint coincident L4.end L5.start
  constraint coincident L16.start origin
  constraint perpendicular L6 L16
  constraint horizontal L17
  constraint vertical L18
  constraint horizontal L19
  constraint vertical L20
  constraint coincident L7.end L8.start
  measures "d45" distance of L4.end L12.end
  measures "d46" distance of L4.end L14.end
  measures "d47" distance of L7.end L17.end
  measures "d48" distance of L7.end L19.end
extrude "Extrude4" cut sketch "Sketch3" against normal blind 10 contours L7 L8 L17 L18 L19 L20
fillet "Fillet3" radius 1 2 edges at (-20.5, 12.5, -10.5) (20.5, 17.5, -10.5)
fillet "Fillet3" radius 1 2 edges at (20.5, 12.5, 10.5) (-20.5, 12.5, 10.5)
fillet "Fillet3" radius 1 2 edges at (25.5, 5, -10.5) (20.5, 5, 5.5)
fillet "Fillet3" radius 1 2 edges at (-35.8, 12.5, -6.5) (35.8, 12.5, -6.5)
fillet "Fillet3" radius 3.5 4 edges at (-35.8, 0, -8.5) (35.8, 0, -8.5) (35.8, 25, -8.5) (-35.8, 25, -8.5)
equation "d19 = ( 23.9 * 2 ) * 1 mm"
equation "d25 = ( 27.8 * 2 ) * 1 mm"
equation "d27 = d25"

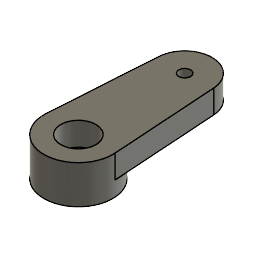
design "attacco motore braccio"
Autodesk Fusion 360 part; units mm, degrees
sketch "Schizzo1" plane through (0, 0, 0) normal (0, 1, 0) x (1, 0, 0)
  circle A0 centre (0, 0) radius 5.9
  line L0 (0, -5.9) -> (0, 22.9)
  line L1 (0, 22.9) -> (0, 18.2)
  circle A1 centre (0, 18.2) radius 4.7
  line L2 (-4.6898, 18.5099) -> (-5.9133, -0.0064)
  line L3 (4.6898, 18.5099) -> (5.9133, -0.0063)
  circle A2 centre (0, 18.2) radius 1
  dimension "d1" = 11.8
  dimension "d2" = 28.8
  dimension "d3" = 4.7
  dimension "d4" = 2
  constraint coincident A0.centre origin
  constraint coincident A0 L0.start
  constraint vertical L0
  constraint parallel L0 L1
  constraint coincident L1.end A1.centre
  constraint coincident L0.end A1
  constraint coincident A1 L2.start
  constraint coincident A1 L3.start
  constraint tangent A1 L3
  constraint tangent A1 L2
  constraint tangent A0 L2
  constraint tangent A0 L3
  constraint concentric A1 A2
  measures "d1" diameter of A0
  measures "d2" distance of L0.start L0.end
  measures "d3" distance of L0.end L1.end
  measures "d4" diameter of A2
extrude "Estrusione1" add sketch "Schizzo1" along normal blind 8.55 contours A0 L0 | A0 L0 | A0 L0 A1 L2 | A0 L0 A1 L3 | L0 L1 A1 A2 | L0 L1 A1 A2
sketch "Schizzo2" plane through (0, 8.55, 0) normal (0, 1, 0) x (-1, 0, 0)
  circle A0 centre (0, -18.2) radius 1
  line L0 (4.6898, -18.5099) -> (5.8872, -0.389)
  arc A1 (5.8872, -0.389) -> (-5.8872, -0.3889) centre (0, 0) ccw
  line L1 (-5.8872, -0.3889) -> (-4.6898, -18.5099)
  arc A2 (-4.6898, -18.5099) -> (4.6898, -18.5099) centre (0, -18.2) ccw
  circle A3 centre (0, 0) radius 3
  dimension "d7" = 6
  constraint coincident A1.centre A3.centre
  measures "d7" diameter of A3
extrude "Estrusione2" cut sketch "Schizzo2" against normal blind 4 contours A3
sketch "Schizzo3" plane through (0, 0, 0) normal (0, -1, 0) x (1, 0, 0)
  circle A0 centre (0, -18.2) radius 1
  line L0 (-5.8872, -0.389) -> (-4.6898, -18.5099)
  arc A1 (-4.6898, -18.5099) -> (4.6898, -18.5099) centre (0, -18.2) ccw
  line L1 (4.6898, -18.5099) -> (5.8872, -0.3889)
  arc A2 (5.8872, -0.3889) -> (-5.8872, -0.389) centre (0, 0) ccw
  circle A3 centre (0, 0) radius 5.9
  line L2 (-5.8998, 0.0466) -> (11.6977, 0.0466)
  line L3 (11.6977, 0.0466) -> (11.6977, -25.1531)
  line L4 (11.6977, -25.1531) -> (-5.8998, -25.1531)
  line L5 (-5.8998, -25.1531) -> (-5.8998, 0.0466)
  circle A4 centre (0, 0) radius 7.5379
  line L6 (0, 0) -> (13.2627, 0)
  line L7 (13.2627, 0) -> (-15, 0)
  constraint coincident A2.centre A3.centre
  constraint horizontal L2
  constraint vertical L3
  constraint horizontal L4
  constraint vertical L5
  constraint coincident A3 L2.start
  constraint coincident A2 L2.start
  constraint concentric A3 A4
  constraint perpendicular L3 L6
  constraint parallel L2 L7
extrude "Estrusione3" cut sketch "Schizzo3" against normal blind 4.55 contours A0 | L0 L1 A3 A4 | L0 A1 L1 A4
extrude "Estrusione5" cut sketch "Schizzo3" against normal blind 2 contours L0 L1 A3 A4 | L0 A2 A3 L5 A4 | A2 A3 L6 L7 | A2 A3 L2 L5 A4 L7 | A2 A3 L2 L5 L6 L7 | L5 A4 L7 | L1 A2 A3 A4 L6 L7 | A2 A3 L2
sketch "Schizzo4" plane through (0, 2, 0) normal (0, -1, 0) x (1, 0, 0)
  circle A0 centre (0, 0) radius 5.9
  circle A1 centre (0, 0) radius 1.5
  dimension "d16" = 3
  constraint coincident A0.centre A1.centre
  measures "d16" diameter of A1
extrude "Estrusione6" cut sketch "Schizzo4" against normal blind 15 contours A1
equation "d3 = ( 9.4 / 2 ) * 1 mm"
equation "d10 = -8.55 mm + 4 mm"
